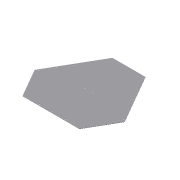
# Autodesk Inventor part: Base Plate
Saved by Autodesk Inventor 2013 (Build 170138000, 138)
## iProperties
Created: 2013-01-11
Part Number: Base Plate
Material: Prefabulated Amulite
Document SubType Name: Modeling
Designer: Naphat
Density: 1 g/cm^3
Author: Naphat
Autodesk Inventor part; units mm, degrees
ref_plane "YZ Plane" through (0, 0, 0) normal (1, 0, 0) x (0, 1, 0)
ref_plane "XZ Plane" through (0, 0, 0) normal (0, 1, 0) x (-1, 0, 0)
ref_plane "XY Plane" through (0, 0, 0) normal (0, 0, 1) x (1, 0, 0)
sketch "Sketch1" plane through (0, 0, 0) normal (0, 1, 0) x (-1, 0, 0)
  line L0 (101.5, -410.6115) -> (-101.7, -410.6115)
  line L1 (101.5, -410.6115) -> (406.3, 117.3176)
  line L2 (406.3, 117.3176) -> (304.7, 293.2939)
  line L3 (304.7, 293.2939) -> (-304.9, 293.2939)
  line L4 (-304.9, 293.2939) -> (-406.5, 117.3176)
  line L5 (-304.9, 293.2939) -> (-101.7, 293.2939) construction
  line L6 (-406.5, 117.3176) -> (-101.7, -410.6115)
  line L7 (-0.1, -410.6115) -> (-0.1, 293.2939) construction
  line L8 (-355.7, 205.3058) -> (253.9, -146.647) construction
  line L9 (-254.1, -146.647) -> (355.5, 205.3058) construction
  line L10 (34.1394, 19.7104) -> (0, 0) construction
  line L11 (0, 0) -> (-34.1644, -19.6671) construction
  line L12 (0, 0) -> (34.1144, -19.7537) construction
  circle A0 centre (-34.1644, -19.6671) radius 3.175 construction
  circle A1 centre (34.1144, -19.7537) radius 3.175 construction
  dimension "d0" = 120
  dimension "d1" = 203.2
  dimension "d3" = 609.6
  dimension "d8" = 203.2
  dimension "d10" = 120
  dimension "d13" = 609.6
  dimension "d15" = 203.2
  dimension "d16" = 120
  dimension "d17" = 609.6
  dimension "d18" = 120
  dimension "d22" = 101.6
  dimension "d122" = 39.4208
  dimension "d123" = 39.4208
  dimension "d124" = 6.35
  dimension "d125" = 6.35
  constraints: 26 end point, 6 midpoint, 2 centre point, 2 coincident, 2 horizontal, 2 parallel, 2 point on line, 1 equal length
  measures "d0" angle of L0 L1
  measures "d1" distance of L0.start L0.end
  measures "d3" distance of L0.start L1.end
  measures "d8" distance of L1.end L2.end
  measures "d10" angle of L1 L2
  measures "d13" distance of L2.end L3.end
  measures "d15" distance of L3.end L4.end
  measures "d16" angle of L4 L5
  measures "d17" distance of L4.end L0.end
  measures "d18" angle of L4 L6
  measures "d22" distance from line of L0.start L7
  measures "d122" distance of L10.end L11.end
  measures "d123" distance of L10.end L12.end
  measures "d124" diameter of A0
  measures "d125" diameter of A1
extrude "Extrusion1" add sketch "Sketch1" against normal blind 1.5
sketch "Sketch2" plane through (0, 0, 0) normal (0, 1, 0) x (1, 0, 0)
  line L0 (-101.5, 410.6115) -> (101.7, 410.6115) projected
  line L1 (-406.3, -117.3176) -> (-101.5, 410.6115) projected
  line L2 (-304.7, -293.2939) -> (-406.3, -117.3176) projected
  line L3 (304.9, -293.2939) -> (-304.7, -293.2939) projected
  line L4 (406.5, -117.3176) -> (304.9, -293.2939) projected
  line L5 (101.7, 410.6115) -> (406.5, -117.3176) projected
  line L6 (0.1, 410.6115) -> (0.1, 350.0579) construction
  line L7 (0.1, 350.0579) -> (136.6606, 350.0579) construction
  line L8 (0.1, 350.0579) -> (-136.4606, 350.0579) construction
  line L9 (-355.5, -205.3058) -> (-303.059, -175.029) construction
  line L10 (355.7, -205.3058) -> (303.259, -175.029) construction
  line L11 (303.259, -175.029) -> (371.5394, -56.764) construction
  line L12 (303.259, -175.029) -> (234.9787, -293.2939) construction
  line L13 (-303.059, -175.029) -> (-234.7787, -293.2939) construction
  line L14 (-303.059, -175.029) -> (-371.3394, -56.764) construction
  line L15 (-371.3394, -56.764) -> (-234.7787, -293.2939)
  line L16 (-304.7, -293.2939) -> (-234.7787, -293.2939)
  line L17 (-304.7, -293.2939) -> (-406.3, -117.3176)
  line L18 (-371.3394, -56.764) -> (-406.3, -117.3176)
  line L19 (-101.5, 410.6115) -> (-136.4606, 350.0579)
  line L20 (-101.5, 410.6115) -> (101.7, 410.6115)
  line L21 (136.6606, 350.0579) -> (101.7, 410.6115)
  line L22 (136.6606, 350.0579) -> (-136.4606, 350.0579)
  line L23 (371.5394, -56.764) -> (234.9787, -293.2939)
  line L24 (304.9, -293.2939) -> (234.9787, -293.2939)
  line L25 (304.9, -293.2939) -> (406.5, -117.3176)
  line L26 (406.5, -117.3176) -> (371.5394, -56.764)
  point P0 (0, 0)
  dimension "d25" = 60.5536
  dimension "d26" = 60.5536
  dimension "d27" = 118.265
  dimension "d28" = 118.265
  dimension "d29" = 118.265
  dimension "d30" = 118.265
  dimension "d31" = 136.5606
  dimension "d32" = 136.5606
  constraints: 42 end point, 14 collinear, 6 perpendicular, 6 point on line, 3 midpoint, 1 parallel
  measures "d25" distance of L6.start L6.end
  measures "d26" distance of L9.start L9.end
  measures "d27" vertical distance of L9.end L14.end
  measures "d28" vertical distance of L9.end L13.end
  measures "d29" vertical distance of L10.end L11.end
  measures "d30" vertical distance of L10.end L12.end
  measures "d31" distance of L6.end L8.end
  measures "d32" distance of L6.end L7.end
extrude "Extrusion2" cut sketch "Sketch2" against normal blind 25.4 contours L0 L5 L22 L1 | L15 L3 L2 L1 | L5 L4 L3 L23
sketch "Sketch5" plane through (0, -1.5, 0) normal (0, -1, 0) x (1, 0, 0)
  line L0 (-234.7787, 293.2939) -> (-371.3394, 56.764) projected
  line L1 (-136.4606, -350.0579) -> (136.6606, -350.0579) projected
  line L2 (136.6606, -350.0579) -> (371.5394, 56.764) projected
  line L3 (371.5394, 56.764) -> (234.9787, 293.2939) projected
  line L4 (-303.059, 175.029) -> (-281.062, 162.329) construction
  line L5 (303.259, 175.029) -> (281.262, 162.329) construction
  line L6 (0.1, -350.0579) -> (0.1, -324.6579) construction
  line L7 (-371.3394, 56.764) -> (-349.3423, 44.064) construction
  line L8 (234.9787, 293.2939) -> (212.9817, 280.5939) construction
  line L9 (371.5394, 56.764) -> (349.5423, 44.064) construction
  line L10 (-136.4606, -350.0579) -> (-136.4606, -324.6579) construction
  line L11 (136.6606, -350.0579) -> (136.6606, -324.6579) construction
  line L12 (-136.4606, -324.6579) -> (-136.4606, -324.6579) construction
  line L13 (136.6606, -324.6579) -> (136.6606, -324.6579) construction
  line L14 (-349.3423, 44.064) -> (-349.3423, 44.064) construction
  line L15 (-234.7787, 293.2939) -> (-212.7817, 280.5939) construction
  line L16 (-212.7817, 280.5939) -> (-212.7817, 280.5939) construction
  circle A0 centre (-349.3423, 44.064) radius 3.175
  circle A1 centre (-212.7817, 280.5939) radius 3.175
  circle A2 centre (212.9817, 280.5939) radius 3.175
  circle A3 centre (349.5423, 44.064) radius 3.175
  circle A4 centre (136.6606, -324.6579) radius 3.175
  circle A5 centre (-136.4606, -324.6579) radius 3.175
  line L17 (212.9817, 280.5939) -> (212.9817, 280.5939)
  line L18 (349.5423, 44.064) -> (349.5423, 44.064)
  line L19 (-212.7817, 280.5939) -> (-106.3408, 280.5939) construction
  line L20 (-106.3408, 280.5939) -> (0.1, 280.5939) construction
  line L21 (0.1, 280.5939) -> (106.5408, 280.5939) construction
  line L22 (106.5408, 280.5939) -> (212.9817, 280.5939) construction
  circle A6 centre (-106.3408, 280.5939) radius 3.175
  circle A7 centre (0.1, 280.5939) radius 3.175
  circle A8 centre (106.5408, 280.5939) radius 3.175
  line L23 (-349.3423, 44.064) -> (-296.1219, -48.1165) construction
  line L24 (-296.1219, -48.1165) -> (-242.9015, -140.297) construction
  line L25 (-242.9015, -140.297) -> (-189.6811, -232.4774) construction
  line L26 (-189.6811, -232.4774) -> (-136.4606, -324.6579) construction
  circle A9 centre (-296.1219, -48.1165) radius 3.175
  circle A10 centre (-242.9015, -140.297) radius 3.175
  circle A11 centre (-189.6811, -232.4774) radius 3.175
  line L27 (136.6606, -324.6579) -> (189.8811, -232.4774) construction
  line L28 (189.8811, -232.4774) -> (243.1015, -140.297) construction
  line L29 (243.1015, -140.297) -> (296.3219, -48.1165) construction
  line L30 (296.3219, -48.1165) -> (349.5423, 44.064) construction
  circle A12 centre (189.8811, -232.4774) radius 3.175
  circle A13 centre (243.1015, -140.297) radius 3.175
  circle A14 centre (296.3219, -48.1165) radius 3.175
  point P0 (0, 0)
  dimension "d67" = 25.4
  dimension "d68" = 25.4
  dimension "d69" = 25.4
  dimension "d70" = 25.4
  dimension "d71" = 25.4
  dimension "d72" = 25.4
  dimension "d73" = 0
  dimension "d74" = 0
  dimension "d75" = 0
  dimension "d76" = 0
  dimension "d77" = 6.35
  dimension "d78" = 6.35
  dimension "d79" = 6.35
  dimension "d80" = 6.35
  dimension "d81" = 6.35
  dimension "d82" = 6.35
  dimension "d83" = 0
  dimension "d84" = 0
  dimension "d87" = 425.7634
  dimension "d88" = 106.4408
  dimension "d89" = 106.4408
  dimension "d90" = 106.4408
  dimension "d91" = 106.4408
  dimension "d92" = 6.35
  dimension "d93" = 6.35
  dimension "d94" = 6.35
  dimension "d95" = 106.4408
  dimension "d96" = 106.4408
  dimension "d97" = 106.4408
  dimension "d98" = 106.4408
  dimension "d99" = 6.35
  dimension "d100" = 6.35
  dimension "d101" = 6.35
  dimension "d102" = 106.4408
  dimension "d103" = 106.4408
  dimension "d104" = 106.4408
  dimension "d105" = 106.4408
  dimension "d106" = 6.35
  dimension "d107" = 6.35
  dimension "d108" = 6.35
  constraints: 54 end point, 15 centre point, 12 coincident, 10 equal length, 7 perpendicular, 3 midpoint, 1 point on line
  measures "d67" distance of L4.start L4.end
  measures "d68" distance of L5.start L5.end
  measures "d69" distance of L6.start L6.end
  measures "d70" distance of L0.end L7.end
  measures "d71" distance of L3.end L8.end
  measures "d72" distance of L2.end L9.end
  measures "d73" distance of L10.end L12.end
  measures "d74" distance of L11.end L13.end
  measures "d75" distance of L7.end L14.end
  measures "d76" distance of L15.end L16.end
  measures "d77" diameter of A0
  measures "d78" diameter of A1
  measures "d79" diameter of A2
  measures "d80" diameter of A3
  measures "d81" diameter of A4
  measures "d82" diameter of A5
  measures "d83" distance of L8.end L17.end
  measures "d84" distance of L9.end L18.end
  measures "d87" distance of L17.end L19.start
  measures "d88" distance of L19.start L19.end
  measures "d89" distance of L19.end L20.end
  measures "d90" distance of L20.end L21.end
  measures "d91" distance of L21.end L17.end
  measures "d92" diameter of A6
  measures "d93" diameter of A7
  measures "d94" diameter of A8
  measures "d95" distance of L23.start L23.end
  measures "d96" distance of L23.end L24.end
  measures "d97" distance of L24.end L25.end
  measures "d98" distance of L25.end L26.end
  measures "d99" diameter of A10
  measures "d100" diameter of A9
  measures "d101" diameter of A11
  measures "d102" distance of L27.start L27.end
  measures "d103" distance of L27.end L28.end
  measures "d104" distance of L28.end L29.end
  measures "d105" distance of L29.end L30.end
  measures "d106" diameter of A12
  measures "d107" diameter of A13
  measures "d108" diameter of A14
extrude "Extrusion5" cut sketch "Sketch5" against normal blind 25.4 contours A0 | A1 | A2 | A3 | A4 | A5
sketch "Sketch6" plane through (0, -1.5, 0) normal (0, -1, 0) x (1, 0, 0)
  circle A0 centre (-106.3408, 280.5939) radius 3.175
  circle A1 centre (0.1, 280.5939) radius 3.175
  circle A2 centre (106.5408, 280.5939) radius 3.175
  circle A3 centre (-296.1219, -48.1165) radius 3.175
  circle A4 centre (-242.9015, -140.297) radius 3.175
  circle A5 centre (-189.6811, -232.4774) radius 3.175
  circle A6 centre (189.8811, -232.4774) radius 3.175
  circle A7 centre (243.1015, -140.297) radius 3.175
  circle A8 centre (296.3219, -48.1165) radius 3.175
  point P0 (0, 0)
  dimension "d109" = 6.35
  dimension "d110" = 6.35
  dimension "d111" = 6.35
  dimension "d112" = 6.35
  dimension "d113" = 6.35
  dimension "d114" = 6.35
  dimension "d115" = 6.35
  dimension "d116" = 6.35
  dimension "d117" = 6.35
  constraints: 9 centre point
  measures "d109" diameter of A0
  measures "d110" diameter of A1
  measures "d111" diameter of A2
  measures "d112" diameter of A4
  measures "d113" diameter of A3
  measures "d114" diameter of A5
  measures "d115" diameter of A6
  measures "d116" diameter of A7
  measures "d117" diameter of A8
extrude "Extrusion6" cut sketch "Sketch6" against normal blind 25.4
sketch "Sketch7" plane through (0, -1.5, 0) normal (0, -1, 0) x (1, 0, 0)
  circle A0 centre (-34.1644, -19.6671) radius 3.175
  circle A1 centre (34.1144, -19.7537) radius 3.175
  point P0 (0, 0)
  dimension "d126" = 6.35
  dimension "d127" = 6.35
  constraints: 2 centre point
  measures "d126" diameter of A0
  measures "d127" diameter of A1
extrude "Extrusion7" cut sketch "Sketch7" against normal blind 25.4
equation "\"d8\" = d1"
equation "\"d13\" = d3"
equation "\"d15\" = d1"
equation "\"d124\" = d125"
equation "\"d88\" = 0.25 * d87"
equation "\"d90\" = d88"
equation "\"d91\" = d88"
equation "\"d92\" = d78"
equation "\"d93\" = d78"
equation "\"d94\" = d78"
equation "\"d95\" = d88"
equation "\"d96\" = d95"
equation "\"d97\" = d96"
equation "\"d98\" = d97"
equation "\"d99\" = d100"
equation "\"d100\" = d77"
equation "\"d101\" = d99"
equation "\"d102\" = d103"
equation "\"d103\" = d104"
equation "\"d104\" = d98"
equation "\"d105\" = d104"
equation "\"d106\" = d107"
equation "\"d107\" = d108"
equation "\"d108\" = d94"
equation "\"d109\" = d118"
equation "\"d110\" = d118"
equation "\"d111\" = d118"
equation "\"d112\" = d113"
equation "\"d113\" = d119"
equation "\"d114\" = d112"
equation "\"d115\" = d116"
equation "\"d116\" = d117"
equation "\"d117\" = d111"
equation "\"d126\" = d127"
equation "\"d118\" = 6.35"
equation "\"d119\" = 6.35"
body "Solid1"
